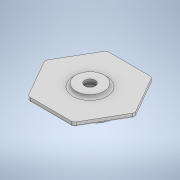
# Autodesk Inventor part: crank case cover
Saved by Autodesk Inventor 2020 (Build 240168000, 168)
## iProperties
Created: 2020-08-07
Part Number: crank case cover
Material: Generic
Document SubType Name: Modeling
Designer: benny
Density: 1 g/cm^3
Appearance: Default
Author: benny
Autodesk Inventor part; units mm, degrees
ref_plane "YZ Plane" through (0, 0, 0) normal (1, 0, 0) x (0, 1, 0)
ref_plane "XZ Plane" through (0, 0, 0) normal (0, 1, 0) x (-1, 0, 0)
ref_plane "XY Plane" through (0, 0, 0) normal (0, 0, 1) x (1, 0, 0)
sketch "Sketch1" plane through (0, 0, 0) normal (0, 1, 0) x (-1, 0, 0)
  circle A0 centre (0, 0) radius 53
  line L0 (-30.4755, 53.0714) -> (30.7235, 52.9283)
  line L1 (30.7235, 52.9283) -> (61.199, -0.1432)
  line L2 (61.199, -0.1432) -> (30.4755, -53.0714)
  line L3 (30.4755, -53.0714) -> (-30.7235, -52.9283)
  line L4 (-30.7235, -52.9283) -> (-61.199, 0.1432)
  line L5 (-61.199, 0.1432) -> (-30.4755, 53.0714)
  point P0 (-45.8372, 26.6073)
  dimension "d0" = 106
  constraints: 12 end point, 2 coincident, 1 midpoint, 16 other
extrude "Extrusion1" add sketch "Sketch1" along normal blind 6
sketch "Sketch2" plane through (0, 6, 0) normal (0, 1, 0) x (1, 0, 0)
  circle A0 centre (0, 0) radius 19
  dimension "d3" = 38
  constraints: 1 centre point, 1 coincident
  measures "d3" diameter of A0
extrude "Extrusion2" add sketch "Sketch2" along normal blind 4
sketch "Sketch3" plane through (0, 10, 0) normal (0, 1, 0) x (1, 0, 0)
  circle A0 centre (0, 0) radius 7
  dimension "d6" = 14
  constraints: 1 centre point, 1 coincident
  measures "d6" diameter of A0
extrude "Extrusion3" cut sketch "Sketch3" against normal blind 10
fillet "Fillet1" radius 4 1 edges at (-19, 6, 0)
sketch "Sketch4" plane through (0, 0, 0) normal (0, -1, 0) x (1, 0, 0)
  circle A0 centre (0, 0) radius 45
  dimension "d10" = 90
  constraints: 1 centre point, 1 coincident
  measures "d10" diameter of A0
extrude "Extrusion4" add sketch "Sketch4" along normal blind 5
sketch "Sketch5" plane through (0, -5, 0) normal (0, -1, 0) x (1, 0, 0)
  circle A0 centre (0, 0) radius 44
  dimension "d13" = 88
  constraints: 1 centre point, 1 coincident
  measures "d13" diameter of A0
extrude "Extrusion5" add sketch "Sketch5" along normal blind 1
sketch "Sketch6" plane through (0, -6, 0) normal (0, -1, 0) x (1, 0, 0)
  circle A0 centre (0, 0) radius 40
  dimension "d16" = 80
  constraints: 1 centre point, 1 coincident
  measures "d16" diameter of A0
extrude "Extrusion6" cut sketch "Sketch6" against normal blind 8
chamfer "Chamfer1" distance 1 angle 45 1 edges at (-44, -5, 0) measured on face at (-44, -5.5, 0)
fillet "Fillet2" radius 2 7 edges at (-40, 2, 0) (-0.124, 0, 52.9999) (45.8372, 0, 26.6073) (-45.9612, 0, 26.3926) (-45.8372, 0, -26.6073) (45.9612, 0, -26.3926) (0.124, 0, -52.9999)
fillet "Fillet3" radius 5 12 edges at (30.3839, 0.5858, -52.3433) (30.7235, 4, -52.9283) (60.5226, 0.5858, 0.1416) (61.199, 4, 0.1432) (-30.4755, 4, -53.0714) (-30.1387, 0.5858, -52.4849) (30.4755, 4, 53.0714) (30.1387, 0.5858, 52.4849) (-30.7235, 4, 52.9283) (-30.3839, 0.5858, 52.3433) (-61.199, 4, -0.1432) (-60.5226, 0.5858, -0.1416)
sketch "Sketch9" plane through (0, 2, 0) normal (0, -1, 0) x (1, 0, 0)
  circle A0 centre (0, 0) radius 19
  dimension "d28" = 38
  constraints: 1 centre point, 1 coincident
  measures "d28" diameter of A0
extrude "Extrusion7" add sketch "Sketch9" along normal blind 6
sketch "Sketch10" plane through (0, -4, 0) normal (0, -1, 0) x (1, 0, 0)
  circle A0 centre (0, 0) radius 14
  dimension "d31" = 28
  constraints: 1 centre point, 1 coincident
  measures "d31" diameter of A0
extrude "Extrusion8" cut sketch "Sketch10" against normal blind 8
fillet "Fillet4" radius 2 1 edges at (-19, 2, 0)
body "Solid1"
